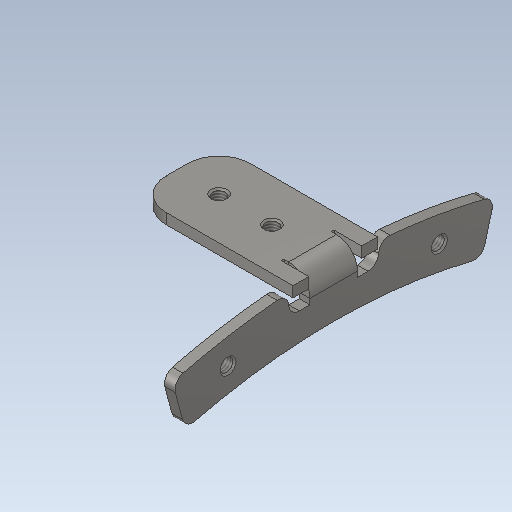
# Autodesk Inventor part: NowyKatownik
Saved by Autodesk Inventor 2020 (Build 240168000, 168)
## iProperties
Created: 2019-05-30
Part Number: NowyKatownik
Material: Stal nierdzewna
Document SubType Name: Konstrukcja blachowa
Designer: barto
Density: 8 g/cm^3
Flat Pattern Width: 3.949 cm
Flat Pattern Length: 6.00698 cm
Flat Pattern Area: 23.7216 cm^2
Sheet Metal Rule: Default_mm
Sheet Metal Width: 39,490 mm
Sheet Metal Length: 60,070 mm
Sheet Metal Area: 2372,156 mm^2
Appearance: Częściowo polerowana
Author: barto
Autodesk Inventor part; units mm, degrees
note: some values were not read from the file. Chosen so that the rebuilt part matches the saved one: relief shape of "Płyta2".
ref_plane "YZ Plane" through (0, 0, 0) normal (1, 0, 0) x (0, 1, 0)
ref_plane "XZ Plane" through (0, 0, 0) normal (0, 1, 0) x (-1, 0, 0)
ref_plane "XY Plane" through (0, 0, 0) normal (0, 0, 1) x (1, 0, 0)
sketch "Szkic1" plane through (0, 0, 0) normal (0, 1, 0) x (-1, 0, 0)
  line L0 (0, 8) -> (-30, 8)
  line L1 (-30, 8) -> (-30, -8)
  line L2 (-30, -8) -> (0, -8)
  line L3 (0, -8) -> (0, 8)
  point P0 (0, 0)
  dimension "d0" = 30
  dimension "d1" = 16
  dimension "d18" = 8
  measures "d0" distance of L1.end L2.end
  measures "d1" distance of L2.end L0.start
  measures "d18" distance from line of point (0, 0) L0
extrude "Płyta1" add sketch "Szkic1" along normal blind 2
sketch "Szkic2" plane through (0, 2, 0) normal (0, 1, 0) x (1, 0, 0)
  line L0 (30, -8) -> (30, 8) projected
  line L1 (30, 5) -> (29.7, 5)
  line L2 (29.7, 5) -> (29.7, -5)
  line L3 (29.7, -5) -> (30, -5)
  line L4 (30, -5) -> (30, 5)
  line L5 (0, 8) -> (30, 8) projected
  point P0 (0, 0)
  dimension "d3" = 10
  dimension "d4" = 3
  dimension "d5" = 0.3
  constraints: 8 end point, 2 parallel, 1 horizontal, 1 perpendicular, 1 point on line, 1 other
  measures "d3" distance of L1.end L2.end
  measures "d5" distance of L1.start L1.end
extrude "Wyciągnięcie proste1" cut sketch "Szkic2" against normal up to next
sketch "Szkic3" plane through (27.7, 2, -5) normal (1, 0, 0) x (0, -1, 0)
  line L0 (0, 9.5) -> (0, 0.5)
  line L1 (0, 0.5) -> (10, 0.5)
  line L2 (10, 0.5) -> (10, 9.5)
  line L3 (10, 9.5) -> (0, 9.5)
  constraints: 8 end point
edge flange "Kołnierz1" height 10 angle 90 thickness 2 bend radius 2 thickness toward (1, 0, 0) relief round relief width 0.5 relief depth 1 edges at (29.7, 2, 0) wall of the first edge with corners at (27.7, 2, 4.5) (27.7, 2, -4.5) (27.7, -8, -4.5) (27.7, -8, 4.5)
bend "Zagięcie1"
corner "Narożnik1"
sketch "Szkic5" plane through (27.7, -8, -4.5) normal (-1, 0, 0) x (0, 0, 1)
  line L0 (9, 0) -> (0, 0)
  arc A0 (32.5897, -3.6981) -> (-23.5897, -3.6981) centre (4.5, -108.5303) ccw
  line L1 (9.5, 10) -> (12.5, 10)
  line L2 (32.5897, -3.6981) -> (34.9889, 5.2557)
  line L3 (-23.5897, -3.6981) -> (-25.9889, 5.2557)
  line L4 (0, 6) -> (9, 6)
  arc A1 (34.9889, 5.2557) -> (13, 8.9626) centre (4.5, -108.5303) ccw
  arc A2 (-4, 8.9626) -> (-25.9889, 5.2557) centre (4.5, -108.5303) ccw
  line L5 (-4, 8.9626) -> (-4, 4.9626)
  line L6 (-4, 4.9626) -> (13, 4.9626)
  line L7 (13, 4.9626) -> (13, 8.9626)
  circle A3 centre (4.5, -108.5303) radius 113
  line L8 (4.5, 0) -> (4.5, -108.5303)
  point P0 (4.5, 8)
  dimension "d38" = 4
  dimension "d39" = 17
  dimension "d42" = 226
  dimension "d69" = 108.5303
  measures "d38" distance of L5.start L5.end
  measures "d39" distance of L5.end L6.end
  measures "d42" diameter of A3
  measures "d69" distance of L8.start L8.end
sheet face with bend "Powierzchnia2" sketch "Szkic5" thickness 2 toward (1, 0, 0) bend radius 2 picked at (25.4474, 0.8245) contours A0 L3 A3 L2 | A3 L3 A2 L5 L6 L7 A1 L2
bend "Zagięcie2"
fillet "Zaokrąglenie narożnika1" radius 2 8 edges at (28.7, 0.9626, -8.5) (28.7, -11.6981, -28.0897) (28.7, -11.6981, 28.0897) (28.7, -3.0374, -8.5) (28.7, -2.7443, 30.4889) (28.7, 0.9626, 8.5) (28.7, -3.0374, 8.5) (28.7, -2.7443, -30.4889)
fillet "Zaokrąglenie narożnika2" radius 6 2 edges at (0, 1, 8) (0, 1, -8)
sketch "Szkic6" plane through (27.7, -2, -4.5) normal (-1, 0, 0) x (0, 0, 1)
  point P0 (4.5, 2)
sketch "Szkic7" plane through (27.7, -2, -4.5) normal (-1, 0, 0) x (0, 0, 1)
  line L0 (9, 0) -> (0, 0) projected
  line L1 (4.5, 0) -> (4.5, -9.6943)
  arc A0 (30.6882, -9.207) -> (-21.6882, -9.207) centre (4.5, -114.5303) ccw projected
  line L2 (4.5, -6) -> (4.5, -114.5303)
  circle A1 centre (4.5, -114.5303) radius 113
  point P0 (4.5, 2)
  point P1 (24.5, -3.3143)
  point P2 (-15.5, -3.3143)
  dimension "d49" = 20
  dimension "d50" = 20
  dimension "d70" = 108.5303
  dimension "d71" = 226
  constraints: 4 end point, 3 point on circle, 2 point on line, 1 centre point, 1 coincident, 1 midpoint, 1 vertical
  measures "d49" distance from line of A1.start L1
  measures "d50" distance from line of L1 A1.end
  measures "d70" distance of L2.start L2.end
  measures "d71" diameter of A1
hole "Otwór1" at (27.7, -5.3143, -20) at (27.7, -5.3143, 20) direction (1, 0, 0) diameter 2.459 end through all thread size "M3x0.5" class "6H" standard "ANSI Metric M Profile"
sketch "Szkic8" plane through (0, 0, 0) normal (0, -1, 0) x (1, 0, 0)
  line L0 (30, 5) -> (30, 8) projected
  point P0 (0, 0)
  point P1 (8, 0)
  point P2 (18, 0)
  dimension "d60" = 8
  dimension "d61" = 10
  dimension "d75" = 12
  measures "d60" distance of point (8, 0) point (0, 0)
  measures "d61" distance of point (18, 0) point (8, 0)
  measures "d75" distance from line of L0 point (18, 0)
hole "Otwór2" at (8, 0, 0) at (18, 0, 0) direction (0, 1, 0) diameter 2.459 end through all thread size "M3x0.5" class "6H" standard "ANSI Metric M Profile"
chamfer "Faza1" distance 0.3 angle 45 4 edges at (29.7, -5.3143, -21.2295) (29.7, -5.3143, 18.7705) (8, 2, 1.2295) (18, 2, 1.2295)
equation "\"d2\" = Grubość"
equation "\"d9\" = GłębokośćGięciaPodcięcia"
equation "\"d10\" = MinimalnaPozostałość"
equation "\"d11\" = PromieńPrzejścia"
equation "\"d14\" = PromieńGięcia"
equation "\"d15\" = RozmiarPodcięciaNarożnika"
equation "\"d16\" = Wielk_odstępu"
equation "\"d17\" = Rozmiar_promienia_Jacobiego"
equation "\"d31\" = PromieńGięcia"
equation "\"d32\" = SzerokośćGięciaPodcięcia"
equation "\"d34\" = MinimalnaPozostałość"
equation "\"d33\" = GłębokośćGięciaPodcięcia"
equation "\"d35\" = PromieńPrzejścia"
equation "\"PromieńGięcia\" = Grubość"
equation "\"SzerokośćGięciaPodcięcia\" = Grubość"
equation "\"GłębokośćGięciaPodcięcia\" = 0.5 * Grubość"
equation "\"RozmiarPodcięciaNarożnika\" = 4 * Grubość"
equation "\"MinimalnaPozostałość\" = 2 * Grubość"
equation "\"PromieńPrzejścia\" = PromieńGięcia"
equation "\"Rozmiar_promienia_Jacobiego\" = PromieńGięcia"
equation "\"Wielk_odstępu\" = Grubość"
equation "\"Grubość\" = 2"
